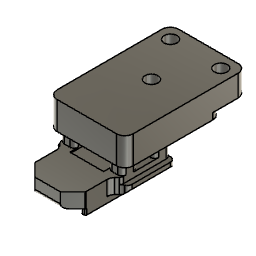
Hybrid_Changer (Autodesk Fusion 360 archive; units mm, degrees)
design "Heating assembly"
Autodesk Fusion 360 part; units mm, degrees
sketch "Sketch1" plane through (0, 0, 0) normal (0, 0, 1) x (1, 0, 0)
  line L0 (9.04, -14.44) -> (-9.04, -14.44)
  line L1 (-9.04, -14.44) -> (-9.04, 14.44)
  line L2 (-9.04, 14.44) -> (9.04, 14.44)
  line L3 (9.04, 14.44) -> (9.04, -14.44)
  line L4 (9.04, -14.44) -> (-9.04, 14.44) construction
  line L5 (-9.04, -14.44) -> (9.04, 14.44) construction
  dimension "d1" = 18.08
  dimension "d2" = 28.88
  constraint horizontal L0
  constraint perpendicular L0 L1
  constraint parallel L0 L2
  constraint parallel L1 L3
  constraint coincident L4 origin
  constraint coincident L5 origin
  measures "d1" distance of L1.end L2.end
  measures "d2" distance of L0.end L1.end
extrude "Extrude1" add sketch "Sketch1" against normal blind 5.6 makes body 1
sketch "Sketch2" plane through (0, 0, 0) normal (0, 0, 1) x (-1, 0, 0)
  line L0 (-9.04, -14.44) -> (9.04, -14.44)
  line L1 (9.04, -14.44) -> (9.04, 14.44)
  line L2 (9.04, 14.44) -> (-9.04, 14.44)
  line L3 (-9.04, 14.44) -> (-9.04, -14.44)
  circle A0 centre (-5.965, -11.415) radius 1.525
  circle A1 centre (5.965, -11.415) radius 1.525
  line L4 (-7.49, -11.415) -> (-9.04, -11.415) construction
  line L5 (-5.965, -12.94) -> (-5.965, -14.44) construction
  line L6 (7.49, -11.415) -> (9.04, -11.415) construction
  line L7 (5.965, -12.94) -> (5.965, -14.44) construction
  circle A2 centre (0, -7.89) radius 1.75
  line L8 (0, -9.64) -> (0, -14.44) construction
  circle A3 centre (0, -0.915) radius 1.525
  line L9 (0, -2.44) -> (0, -0.915) construction
  circle A4 centre (5.89, 11.44) radius 1.85
  circle A5 centre (5.89, 3.44) radius 1.85
  circle A6 centre (-5.89, 11.44) radius 1.85
  circle A7 centre (-5.89, 3.44) radius 1.85
  line L10 (5.89, 13.29) -> (5.89, 11.44) construction
  line L11 (5.89, 11.44) -> (7.74, 11.44) construction
  line L12 (-5.89, 11.44) -> (-7.74, 11.44) construction
  line L13 (5.89, 3.44) -> (5.89, 5.29) construction
  circle A8 centre (5.89, 11.44) radius 1.25
  circle A9 centre (5.89, 3.44) radius 1.25
  circle A10 centre (-5.89, 3.44) radius 1.25
  circle A11 centre (-5.89, 11.44) radius 1.25
  dimension "d5" = 3.05
  dimension "d6" = 1.55
  dimension "d7" = 1.5
  dimension "d8" = 3.5
  dimension "d9" = 4.8
  dimension "d10" = 12
  dimension "d11" = 3.7
  dimension "d12" = 3.7
  dimension "d13" = 3.7
  dimension "d14" = 3.7
  dimension "d15" = 1.15
  dimension "d16" = 1.3
  dimension "d17" = 1.3
  dimension "d18" = 9.15
  dimension "d22" = 2.5
  constraint equal A0 A1
  constraint horizontal A0.centre A1.centre
  constraint coincident A0 L4.start
  constraint coincident L3 L4.end
  constraint perpendicular L3 L4
  constraint coincident A0 L5.start
  constraint coincident L0 L5.end
  constraint perpendicular L0 L5
  constraint coincident A1 L6.start
  constraint coincident L1 L6.end
  constraint perpendicular L1 L6
  constraint coincident A1 L7.start
  constraint coincident L0 L7.end
  constraint perpendicular L0 L7
  constraint horizontal A1.centre L6.start
  constraint vertical A1.centre L7.start
  constraint vertical A0.centre L5.start
  constraint horizontal A0.centre L4.start
  constraint equal L4 L6
  constraint vertical origin A2.centre
  constraint coincident A2 L8.start
  constraint midpoint L0 L8.end
  constraint vertical A2.centre L8.start
  constraint vertical origin A3.centre
  constraint equal A0 A3
  constraint coincident A3 L9.start
  constraint coincident A3.centre L9.end
  constraint vertical L9
  constraint horizontal A4.centre A6.centre
  constraint vertical A4.centre A5.centre
  constraint vertical A6.centre A7.centre
  constraint horizontal A5.centre A7.centre
  constraint coincident A4 L10.start
  constraint coincident A4.centre L10.end
  constraint coincident A4 L11.end
  constraint perpendicular L10 L11
  constraint coincident A6.centre L12.start
  constraint coincident A6 L12.end
  constraint parallel L11 L12
  constraint vertical L10
  constraint coincident A5.centre L13.start
  constraint coincident A5 L13.end
  constraint vertical L13
  constraint concentric A4 A8
  constraint concentric A5 A9
  constraint concentric A7 A10
  constraint concentric A6 A11
  constraint equal A8 A9
  constraint equal A8 A10
  constraint equal A8 A11
  measures "d5" diameter of A0
  measures "d6" distance of L4.start L4.end
  measures "d7" distance of L5.start L5.end
  measures "d8" diameter of A2
  measures "d9" distance of L8.start L8.end
  measures "d10" distance of L8.end L9.start
  measures "d11" diameter of A4
  measures "d12" diameter of A5
  measures "d13" diameter of A6
  measures "d14" diameter of A7
  measures "d15" distance of L2 L10.start
  measures "d16" distance of L1 L11.end
  measures "d17" distance of L3 L12.end
  measures "d18" distance of L2 L13.end
  measures "d22" diameter of A8
extrude "Extrude2" cut sketch "Sketch2" against normal through all contours A0 | A1 | A2 | A3 | A8 | A9 | A10 | A11 bodies 1
extrude "Extrude3" cut sketch "Sketch2" against normal blind 2.35 contours A4 | A5 | A6 | A7 | A8 | A9 | A10 | A11 bodies 1
sketch "Sketch3" plane through (0, 0, -5.6) normal (0, 0, -1) x (1, 0, 0)
  circle A0 centre (-5.89, 11.44) radius 1.25
  circle A1 centre (0, -7.89) radius 1.75
  circle A2 centre (-5.965, -11.415) radius 1.525
  circle A3 centre (5.89, 11.44) radius 1.25
  circle A4 centre (-5.89, 3.44) radius 1.25
  circle A5 centre (0, -0.915) radius 1.525
  circle A6 centre (5.965, -11.415) radius 1.525
  circle A7 centre (5.89, 3.44) radius 1.25
  line L0 (-9.04, -14.44) -> (9.04, -14.44)
  line L1 (9.04, -14.44) -> (9.04, 14.44)
  line L2 (9.04, 14.44) -> (-9.04, 14.44)
  line L3 (-9.04, 14.44) -> (-9.04, -14.44)
  circle A8 centre (0, -0.915) radius 3
  circle A9 centre (5.965, -11.415) radius 3
  circle A10 centre (-5.965, -11.415) radius 3
  line L4 (5.965, -8.415) -> (9.04, -8.415)
  line L5 (2.965, -11.415) -> (2.965, -14.44)
  line L6 (-2.965, -11.415) -> (-2.965, -14.44)
  line L7 (-5.965, -8.415) -> (-9.04, -8.415)
  dimension "d23" = 6
  dimension "d24" = 6
  dimension "d25" = 6
  constraint concentric A5 A8
  constraint concentric A6 A9
  constraint concentric A2 A10
  constraint coincident A9 L4.start
  constraint coincident L1 L4.end
  constraint perpendicular L1 L4
  constraint coincident A9 L5.start
  constraint coincident L0 L5.end
  constraint perpendicular L0 L5
  constraint coincident A10 L6.start
  constraint coincident L0 L6.end
  constraint perpendicular L0 L6
  constraint coincident L3 L7.end
  constraint perpendicular L3 L7
  constraint vertical A6.centre L4.start
  constraint horizontal A6.centre L5.start
  constraint horizontal A2.centre L6.start
  constraint vertical A2.centre L7.start
  constraint coincident A10 L7.start
  measures "d23" diameter of A8
  measures "d24" diameter of A9
  measures "d25" diameter of A10
extrude "Extrude4" cut sketch "Sketch3" against normal blind 1.5 contours A0 | A1 | A2 | A3 | A4 | A5 | A7 | L0 L3 A10 L6 L7 | L0 L1 A9 L4 L5 | A10 | A9 | A8 bodies 1
fillet "Fillet1" radius 2 6 edges at (-9.04, 14.44, -2.05) (9.04, 14.44, -2.05) (-9.04, -14.44, -2.8) (9.04, -14.44, -2.8) (9.04, 8.415, -4.85) (-9.04, 8.415, -4.85) on bodies 1
sketch "Sketch5" plane through (0, 0, -5.6) normal (0, 0, -1) x (1, 0, 0)
  arc A0 (9.04, 12.44) -> (7.04, 14.44) centre (7.04, 12.44) ccw
  line L0 (7.04, 14.44) -> (-7.04, 14.44)
  arc A1 (-7.04, 14.44) -> (-9.04, 12.44) centre (-7.04, 12.44) ccw
  line L1 (-9.04, 12.44) -> (-9.04, -6.415)
  arc A2 (-2.965, -11.415) -> (-5.965, -8.415) centre (-5.965, -11.415) ccw
  line L2 (-2.965, -11.415) -> (-2.965, -14.44)
  line L3 (-2.965, -14.44) -> (2.965, -14.44)
  line L4 (2.965, -14.44) -> (2.965, -11.415)
  arc A3 (5.965, -8.415) -> (2.965, -11.415) centre (5.965, -11.415) ccw
  line L5 (9.04, -6.415) -> (9.04, 12.44)
  circle A4 centre (0, -0.915) radius 3
  circle A5 centre (-5.89, 11.44) radius 1.25
  circle A6 centre (0, -7.89) radius 1.75
  circle A7 centre (5.89, 11.44) radius 1.25
  circle A8 centre (-5.89, 3.44) radius 1.25
  circle A9 centre (5.89, 3.44) radius 1.25
  line L6 (7.34, 1.94) -> (-7.34, 1.94)
  line L7 (-7.34, 1.94) -> (-7.34, 13.44)
  line L8 (-7.34, 13.44) -> (7.34, 13.44)
  line L9 (7.34, 13.44) -> (7.34, 1.94)
  line L10 (7.34, 1.94) -> (-7.34, 13.44) construction
  line L11 (-7.34, 1.94) -> (7.34, 13.44) construction
  line L12 (5.965, -8.415) -> (7.04, -8.415)
  line L13 (-7.04, -8.415) -> (-5.965, -8.415)
  arc A10 (-9.04, -6.415) -> (-7.04, -8.415) centre (-7.04, -6.415) ccw
  arc A11 (7.04, -8.415) -> (9.04, -6.415) centre (7.04, -6.415) ccw
  point P0 (0, 7.69)
  dimension "d33" = 1.7
  dimension "d34" = 1
  dimension "d35" = 12.5
  constraint horizontal L6
  constraint perpendicular L6 L7
  constraint parallel L6 L8
  constraint parallel L7 L9
  constraint coincident L10 P0
  constraint coincident L11 P0
  constraint vertical origin P0
  measures "d33" distance of L5 L9
  measures "d34" distance of L0 L8
  measures "d35" distance of L0 L6
extrude "Extrude5" add sketch "Sketch5" along normal blind 6.2 separate body contours A4 L6 | A4 L6 L7 L8 L9 picked at (0.1862, 1.9708) makes body 2
sketch "Sketch6" plane through (0, 0, -11.8) normal (0, 0, -1) x (1, 0, 0)
  circle A0 centre (5.89, 11.44) radius 1.25
  circle A1 centre (-5.89, 3.44) radius 1.25
  circle A2 centre (5.89, 3.44) radius 1.25
  circle A3 centre (-5.89, 11.44) radius 1.25
  line L0 (7.34, 13.44) -> (-7.34, 13.44)
  line L1 (-7.34, 13.44) -> (-7.34, 1.94)
  line L2 (-7.34, 1.94) -> (7.34, 1.94)
  line L3 (7.34, 1.94) -> (7.34, 13.44)
  line L4 (8.5, 1.94) -> (-8.5, 1.94)
  line L5 (-8.5, 1.94) -> (-8.5, 12.94)
  line L6 (-8.5, 12.94) -> (8.5, 12.94)
  line L7 (8.5, 12.94) -> (8.5, 1.94)
  line L8 (8.5, 1.94) -> (-8.5, 12.94) construction
  line L9 (-8.5, 1.94) -> (8.5, 12.94) construction
  line L10 (8.5, 12.94) -> (7.34, 13.44)
  line L11 (-7.34, 13.44) -> (-8.5, 12.94)
  point P0 (0, 7.44)
  dimension "d38" = 17
  dimension "d39" = 11
  constraint horizontal L4
  constraint perpendicular L4 L5
  constraint parallel L4 L6
  constraint parallel L5 L7
  constraint coincident L8 P0
  constraint coincident L9 P0
  constraint vertical origin P0
  constraint coincident L2.end L4
  constraint coincident L0.start L3.end
  constraint coincident L0.end L1.start
  measures "d38" distance of L5.end L6.end
  measures "d39" distance of L4.end L5.end
extrude "Extrude6" add sketch "Sketch6" against normal blind 2 contours A0 | A1 | A2 | A3 | L3 L6 L10 | L1 L6 L11 | L3 L4 L6 L7 | L1 L2 L3 L4 L6 | L1 L4 L5 L6 bodies 2
sketch "Sketch7" plane through (0, 0, -11.8) normal (0, 0, -1) x (1, 0, 0)
  line L0 (7.34, 13.44) -> (-7.34, 13.44)
  line L1 (-8.5, 12.94) -> (-8.5, 1.94)
  line L2 (-8.5, 1.94) -> (8.5, 1.94)
  line L3 (8.5, 1.94) -> (8.5, 12.94)
  line L4 (6.025, 13.44) -> (-6.025, 13.44)
  line L5 (-6.025, 13.44) -> (-6.025, 23.74)
  line L6 (-6.025, 23.74) -> (6.025, 23.74)
  line L7 (6.025, 23.74) -> (6.025, 13.44)
  line L8 (0, 23.74) -> (0, 0) construction
  line L9 (8.5, 12.94) -> (7.34, 13.44)
  line L10 (-7.34, 13.44) -> (-8.5, 12.94)
  line L11 (7.34, 13.44) -> (6.025, 14.94)
  line L12 (-6.025, 14.94) -> (-7.34, 13.44)
  dimension "d42" = 12.05
  dimension "d43" = 10.3
  dimension "d70" = 1.5
  constraint horizontal L4
  constraint vertical L5
  constraint horizontal L6
  constraint vertical L7
  constraint coincident L0 L4.start
  constraint midpoint L6 L8.start
  constraint coincident L8.end origin
  constraint vertical L8
  constraint coincident L0.start L9.end
  constraint coincident L7 L11.end
  constraint coincident L5 L12.start
  constraint coincident L0.end L10.start
  constraint horizontal L11.end L12.start
  measures "d42" distance of L4.start L4.end
  measures "d43" distance of L4.start L6.end
  measures "d70" distance of L4.start L11.end
extrude "Extrude7" add sketch "Sketch7" against normal blind 3.5 contours L0 L7 L11 | L0 L4 L5 L6 L7 | L0 L5 L12 bodies 2
chamfer "Chamfer3" distance 3 angle 45 2 edges at (6.025, -23.74, -10.05) (-6.025, -23.74, -10.05) on bodies 2
sketch "Sketch10" plane through (0, 0, -11.8) normal (0, 0, -1) x (1, 0, 0)
  line L0 (-6.025, 20.74) -> (-6.025, 14.94)
  line L1 (-8.5, 12.94) -> (-8.5, 1.94)
  line L2 (-8.5, 1.94) -> (8.5, 1.94)
  line L3 (8.5, 1.94) -> (8.5, 12.94)
  line L4 (6.025, 14.94) -> (6.025, 20.74)
  line L5 (3.025, 23.74) -> (-3.025, 23.74)
  line L6 (6.025, 20.74) -> (5.025, 20.74)
  line L7 (5.025, 20.74) -> (5.025, 1.94)
  line L8 (5.025, 1.94) -> (6.025, 1.94)
  line L9 (6.025, 1.94) -> (6.025, 20.74)
  line L10 (-6.025, 20.74) -> (-5.025, 20.74)
  line L11 (-5.025, 20.74) -> (-5.025, 1.94)
  line L12 (-5.025, 1.94) -> (-6.025, 1.94)
  line L13 (-6.025, 1.94) -> (-6.025, 3.24)
  line L14 (-6.525, 3.74) -> (-7.025, 3.74)
  line L15 (-7.025, 3.74) -> (-7.025, 11.64)
  line L16 (-7.025, 11.64) -> (-6.525, 11.64)
  line L17 (-6.025, 11.64) -> (-6.025, 3.74)
  arc A0 (-6.025, 3.24) -> (-6.525, 3.74) centre (-6.525, 3.24) ccw
  line L18 (-6.025, 14.94) -> (-6.025, 12.14)
  arc A1 (-6.525, 11.64) -> (-6.025, 12.14) centre (-6.525, 12.14) ccw
  line L19 (-3.025, 23.74) -> (-6.025, 20.74)
  line L20 (6.025, 20.74) -> (3.025, 23.74)
  line L21 (7.34, 13.44) -> (8.5, 12.94)
  line L22 (8.5, 12.94) -> (7.34, 13.44)
  line L23 (-7.34, 13.44) -> (-8.5, 12.94)
  line L24 (-6.025, 14.94) -> (-7.34, 13.44)
  line L25 (7.34, 13.44) -> (6.025, 14.94)
  dimension "d55" = 1
  dimension "d56" = 1
  dimension "d60" = 1
  dimension "d61" = 1.8
  dimension "d63" = 0.5
  dimension "d64" = 0.5
  constraint horizontal L6
  constraint vertical L7
  constraint horizontal L8
  constraint vertical L9
  constraint coincident L4.end L6.start
  constraint horizontal L10
  constraint vertical L11
  constraint horizontal L12
  constraint vertical L13
  constraint coincident L2 L11.end
  constraint coincident L0.start L10.start
  constraint coincident L2 L7.end
  constraint horizontal L14
  constraint vertical L15
  constraint horizontal L16
  constraint vertical L17
  constraint coincident L13 L17.end
  constraint coincident L17.end L14
  constraint coincident L0.start L13
  constraint tangent L14 A0
  constraint tangent L13 A0
  constraint coincident L0.end L18.start
  constraint coincident L17.start L16
  constraint coincident L17.start L18
  constraint tangent L16 A1
  constraint tangent L18 A1
  constraint coincident L21.start L22.end
  constraint coincident L3.end L21.end
  measures "d55" distance of L4.end L6.end
  measures "d56" distance of L0.start L10.end
  measures "d60" distance of L17.end L14.end
  measures "d61" distance of L2 L14
  measures "d63" radius of A0
  measures "d64" radius of A1
extrude "Extrude10" add sketch "Sketch10" along normal blind 1.65 contours L0 L2 L10 L11 L12 L13 L14 L15 L16 A0 L18 A1 | L2 L4 L6 L7 L8 L9 bodies 2
chamfer "Chamfer2" distance 1 angle 45 2 edges at (8.5, -7.44, -11.8) (-8.5, -7.44, -11.8) on bodies 2
sketch "Sketch11" plane through (0, 0, -11.8) normal (0, 0, -1) x (1, 0, 0)
  line L0 (7.5, 1.94) -> (7.5, 13.371)
  line L1 (6.025, 14.94) -> (6.025, 1.94)
  line L2 (6.025, 1.94) -> (7.5, 1.94)
  line L3 (6.025, 1.94) -> (6.025, 20.74)
  line L4 (7.5, 13.371) -> (7.34, 13.44)
  line L5 (7.34, 13.44) -> (6.025, 14.94)
  point P0 (8.5, 12.94)
  point P1 (8.5, 1.94)
fillet "Fillet3" radius 1.15 4 edges at (-8.5, -12.94, -10.3) (8.5, -12.94, -10.3) (8.5, -1.94, -10.3) (-8.5, -1.94, -10.3) on bodies 2
fillet "Fillet4" radius 2 4 edges at (6.025, -14.94, -10.05) (7.34, -13.44, -10.8) (-6.025, -14.94, -10.05) (-7.34, -13.44, -10.8) on bodies 2
sketch "Sketch12" plane through (7.34, 0, 0) normal (1, 0, 0) x (0, 1, 0)
  line L0 (-13.5027, -9.8) -> (-1.94, -9.8)
  line L1 (-1.94, -9.8) -> (-1.94, -5.6)
  line L2 (-1.94, -5.6) -> (-13.44, -5.6)
  line L3 (-13.44, -5.6) -> (-13.44, -8.3)
  line L4 (-13.44, -8.3) -> (-13.5027, -8.3)
  line L5 (-13.5027, -8.3) -> (-13.5027, -9.8)
  line L6 (-5.69, -5.6) -> (-9.69, -5.6)
  line L7 (-9.69, -5.6) -> (-9.69, -8.6)
  line L8 (-9.69, -8.6) -> (-5.69, -8.6)
  line L9 (-5.69, -8.6) -> (-5.69, -5.6)
  point P0 (-7.69, -5.6)
  point P1 (-7.69, -8.6)
  dimension "d73" = 4
  dimension "d74" = 3
  constraint horizontal L6
  constraint vertical L7
  constraint horizontal L8
  constraint vertical L9
  constraint coincident L2 L6.start
  constraint midpoint L2 P0
  constraint midpoint L8 P1
  constraint vertical P0 P1
  measures "d73" distance of L6.start L6.end
  measures "d74" distance of L6.start L8.end
extrude "Extrude11" cut sketch "Sketch12" against normal through all contours L2 L6 L7 L8 L9 bodies 2
sketch "Sketch13" plane through (0, -1.94, 0) normal (0, 1, 0) x (-1, 0, 0)
  line L0 (7.35, -11.8) -> (7.35, -9.8)
  line L1 (7.35, -9.8) -> (7.34, -9.8)
  line L2 (7.34, -9.8) -> (7.34, -5.6)
  line L3 (7.34, -5.6) -> (-7.34, -5.6)
  line L4 (-7.34, -5.6) -> (-7.34, -9.8)
  line L5 (-7.34, -9.8) -> (-7.35, -9.8)
  line L6 (-7.35, -9.8) -> (-7.35, -11.8)
  line L7 (-7.35, -11.8) -> (-6.025, -11.8)
  line L8 (-6.025, -11.8) -> (-6.025, -13.45)
  line L9 (-6.025, -13.45) -> (-5.025, -13.45)
  line L10 (-5.025, -13.45) -> (-5.025, -11.8)
  line L11 (-5.025, -11.8) -> (5.025, -11.8)
  line L12 (5.025, -11.8) -> (5.025, -13.45)
  line L13 (5.025, -13.45) -> (6.025, -13.45)
  line L14 (6.025, -13.45) -> (6.025, -11.8)
  line L15 (6.025, -11.8) -> (7.35, -11.8)
  line L16 (4, -5.6) -> (-4, -5.6)
  line L17 (-4, -5.6) -> (-4, -8.6)
  line L18 (-4, -8.6) -> (4, -8.6)
  line L19 (4, -8.6) -> (4, -5.6)
  point P0 (0, -5.6)
  point P1 (0, -8.6)
  dimension "d76" = 8
  dimension "d77" = 3
  constraint horizontal L16
  constraint vertical L17
  constraint horizontal L18
  constraint vertical L19
  constraint coincident L3 L16.start
  constraint midpoint L3 P0
  constraint midpoint L18 P1
  constraint vertical P0 P1
  measures "d76" distance of L16.start L16.end
  measures "d77" distance of L16.start L18.end
extrude "Extrude12" cut sketch "Sketch13" against normal blind 12.5 contours L3 L16 L17 L18 L19 bodies 2
fillet "Fillet5" radius 1 19 edges at (-7.34, -1.94, -7.7) (-7.34, -5.69, -7.1) (-4, -1.94, -7.1) (-4, -5.69, -7.1) (-7.34, -9.69, -7.1) (-4, -9.69, -7.1) (-7.34, -13.44, -6.95) (-4, -13.44, -6.95) (4, -1.94, -7.1) (7.34, -1.94, -7.7) (4, -5.69, -7.1) (7.34, -5.69, -7.1) (4, -9.69, -7.1) (7.34, -9.69, -7.1) (7.34, -13.44, -6.95) (4, -13.44, -6.95) (7.34, -13.5027, -9.05) (-7.34, -13.5027, -9.05) (0, -23.74, -11.8) on bodies 2
fillet "Fillet6" radius 0.25 23 edges at (5.025, -20.74, -12.625) (6.025, -11.34, -13.45) (5.525, -20.74, -13.45) (5.025, -11.34, -13.45) (-5.025, -20.74, -12.625) (-6.025, -20.74, -12.625) (-6.025, -20.74, -10.05) (6.025, -20.74, -12.625) (6.025, -20.74, -10.05) (-5.025, -11.34, -13.45) (-5.525, -20.74, -13.45) (-6.025, -16.44, -13.45) (-6.1714, -11.7864, -13.45) (-6.775, -11.64, -13.45) (-6.775, -3.74, -13.45) (-6.1714, -3.5936, -13.45) (-6.025, -2.59, -13.45) (6.025, -1.94, -12.625) (5.025, -1.94, -12.625) (-6.025, -1.94, -12.625) (-5.025, -1.94, -12.625) (-7.025, -11.64, -12.625) (-7.025, -3.74, -12.625) on bodies 2
sketch "Sketch14" plane through (0, 0, 0) normal (0, 0, 1) x (-1, 0, 0)
  circle A0 centre (5.89, 11.44) radius 1.85
  circle A1 centre (-5.89, 11.44) radius 1.85
  circle A2 centre (5.89, 3.44) radius 1.85
  circle A3 centre (-5.89, 3.44) radius 1.85
  circle A4 centre (0, -7.89) radius 1.75
  circle A5 centre (5.965, -11.415) radius 1.525
  circle A6 centre (0, -0.915) radius 1.525
  circle A7 centre (-5.965, -11.415) radius 1.525
  arc A8 (-7.04, 14.44) -> (-9.04, 12.44) centre (-7.04, 12.44) ccw
  line L0 (-9.04, 12.44) -> (-9.04, -12.44)
  arc A9 (-9.04, -12.44) -> (-7.04, -14.44) centre (-7.04, -12.44) ccw
  line L1 (-7.04, -14.44) -> (7.04, -14.44)
  arc A10 (7.04, -14.44) -> (9.04, -12.44) centre (7.04, -12.44) ccw
  line L2 (9.04, -12.44) -> (9.04, 12.44)
  arc A11 (9.04, 12.44) -> (7.04, 14.44) centre (7.04, 12.44) ccw
  line L3 (7.04, 14.44) -> (-7.04, 14.44)
extrude "Extrude13" add sketch "Sketch14" along normal blind 5 separate body makes body 3
sketch "Sketch15" plane through (0, 0, 5) normal (0, 0, 1) x (-1, 0, 0)
  circle A0 centre (5.89, 11.44) radius 1.85
  circle A1 centre (5.89, 3.44) radius 1.85
  circle A2 centre (-5.89, 11.44) radius 1.85
  circle A3 centre (-5.89, 3.44) radius 1.85
  circle A4 centre (0, -0.915) radius 1.525
  circle A5 centre (0, -7.89) radius 1.75
  circle A6 centre (-5.965, -11.415) radius 1.525
  circle A7 centre (5.965, -11.415) radius 1.525
  line L0 (7.04, 14.44) -> (-7.04, 14.44)
  arc A8 (-7.04, 14.44) -> (-9.04, 12.44) centre (-7.04, 12.44) ccw
  line L1 (-9.04, 12.44) -> (-9.04, -12.44)
  arc A9 (-9.04, -12.44) -> (-7.04, -14.44) centre (-7.04, -12.44) ccw
  line L2 (-7.04, -14.44) -> (7.04, -14.44)
  arc A10 (7.04, -14.44) -> (9.04, -12.44) centre (7.04, -12.44) ccw
  line L3 (9.04, -12.44) -> (9.04, 12.44)
  arc A11 (9.04, 12.44) -> (7.04, 14.44) centre (7.04, 12.44) ccw
  circle A12 centre (5.965, -11.415) radius 2.1
  circle A13 centre (0, -0.915) radius 2.1
  circle A14 centre (-5.965, -11.415) radius 2.1
  dimension "d86" = 4.2
  dimension "d87" = 4.2
  dimension "d88" = 4.2
  constraint concentric A7 A12
  constraint concentric A4 A13
  constraint concentric A6 A14
  measures "d86" diameter of A12
  measures "d87" diameter of A13
  measures "d88" diameter of A14
extrude "Extrude14" cut sketch "Sketch15" against normal blind 11 contours A12 | A13 | A14 bodies 3
copy_body "Body->Comp1" bodies 3 removing the originals makes body 4 in component "Component"
sketch "Sketch16" plane through (0, 0, 0) normal (0, 0, 1) x (-1, 0, 0)
  arc A0 (-7.04, 14.44) -> (-9.04, 12.44) centre (-7.04, 12.44) ccw
  line L0 (-9.04, 12.44) -> (-9.04, -12.44)
  arc A1 (-9.04, -12.44) -> (-7.04, -14.44) centre (-7.04, -12.44) ccw
  line L1 (-7.04, -14.44) -> (7.04, -14.44)
  arc A2 (7.04, -14.44) -> (9.04, -12.44) centre (7.04, -12.44) ccw
  line L2 (9.04, -12.44) -> (9.04, 12.44)
  arc A3 (9.04, 12.44) -> (7.04, 14.44) centre (7.04, 12.44) ccw
  line L3 (7.04, 14.44) -> (-7.04, 14.44)
  circle A4 centre (5.89, 11.44) radius 1.85
  circle A5 centre (-5.89, 11.44) radius 1.85
  circle A6 centre (5.89, 3.44) radius 1.85
  circle A7 centre (-5.89, 3.44) radius 1.85
  circle A8 centre (0, -7.89) radius 1.75
  circle A9 centre (5.965, -11.415) radius 1.525
  circle A10 centre (0, -0.915) radius 1.525
  circle A11 centre (-5.965, -11.415) radius 1.525
extrude "Extrude15" add sketch "Sketch16" along normal blind 1 contours A0 L0 A1 L1 A2 L2 A3 L3 | A4 | A5 | A6 | A7 | A8 bodies 1
sketch "Sketch17" plane through (0, 0, 1) normal (0, 0, 1) x (-1, 0, 0)
  circle A0 centre (0, -0.915) radius 1.525
  circle A1 centre (5.965, -11.415) radius 1.525
  circle A2 centre (-5.965, -11.415) radius 1.525
  line L0 (7.04, 14.44) -> (-7.04, 14.44)
  arc A3 (-7.04, 14.44) -> (-9.04, 12.44) centre (-7.04, 12.44) ccw
  line L1 (-9.04, 12.44) -> (-9.04, -12.44)
  arc A4 (-9.04, -12.44) -> (-7.04, -14.44) centre (-7.04, -12.44) ccw
  line L2 (-7.04, -14.44) -> (7.04, -14.44)
  arc A5 (7.04, -14.44) -> (9.04, -12.44) centre (7.04, -12.44) ccw
  line L3 (9.04, -12.44) -> (9.04, 12.44)
  arc A6 (9.04, 12.44) -> (7.04, 14.44) centre (7.04, 12.44) ccw
component "Component" placed x (1, 0, 0) y (0, 1, 0) z (0, 0, 1) at (0, 0, 0)
equation "d17 = d16"

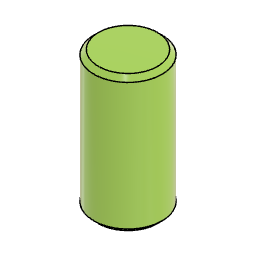
design "Steel_rod_6mm"
Autodesk Fusion 360 part; units mm, degrees
sketch "Sketch1" plane through (0, 0, 0) normal (0, 0, 1) x (1, 0, 0)
  circle A0 centre (0, 0) radius 1.5
  dimension "d1" = 3
  constraint coincident A0.centre origin
  measures "d1" diameter of A0
extrude "Extrude1" add sketch "Sketch1" along normal blind 6 makes body 1
chamfer "Chamfer1" distance 0.2 angle 45 2 edges at (-1.3985, -0.5424, 6) (-1.3985, -0.5424, 0) on bodies 1
copy_body "Body->Comp1" bodies 1 removing the originals makes body 2 in component "Component"
component "Component" placed x (1, 0, 0) y (0, 1, 0) z (0, 0, 1) at (0, 0, 0)
equation "d2 = Length"
equation "Length = 6 mm"

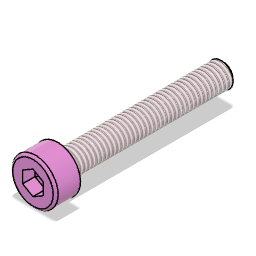
design "Broached Hexagon Socket Head Cap Screw ANSI B18.3.1M - M3x0.5 x 20 Steel Grade 2 Plain"
description: Broached Hexagon Socket Head Cap Screw ANSI B18.3.1M - M3x0.5 x 20
Autodesk Fusion 360 part; units mm, degrees
sketch "Sketch1" plane through (0, 0, 0) normal (0, 1, 0) x (1, 0, 0)
  line L0 (-1.5, 0) -> (-1.5, 20)
  line L1 (-1.5, 20) -> (0, 20)
  line L2 (0, 20) -> (0, -3)
  line L3 (-1.5, 0) -> (-2.75, 0)
  line L4 (-2.75, 0) -> (-2.75, -3)
  line L5 (-2.75, -3) -> (0, -3)
  dimension "d9" = 3
  dimension "d66" = 5.5
  dimension "d68" = 20
  dimension "d79" = 3
  constraint perpendicular L0 L1
  constraint collinear origin L1.end L2.end
  constraint perpendicular L0 L3
  constraint coincident origin L3
  constraint vertical L0
  constraint vertical L2
  constraint parallel L2 L4
  constraint coincident L2 L5.end
  constraint perpendicular L2 L5
  measures "d68" distance of origin L1.end
  measures "d79" distance of L3.end L4.end
revolve "Revolve1" add sketch "Sketch1" angle 360 about axis through (0, 0, -20) along (0, 0, 1)
ref_plane "WorkPlane1" through (0, 0, 3) normal (0, 0, 1) x (1, 0, 0)
sketch "Sketch6" plane through (0, 0, 3) normal (0, 0, 1) x (1, 0, 0)
  line L0 (-1.25, 0) -> (1.25, 0) construction
  line L1 (0, 0) -> (-1.25, 0.7217)
  line L2 (-1.25, -0.7217) -> (-1.25, 0.7217)
  line L3 (-1.25, -0.7217) -> (0, 0)
  dimension "d72" = 2.5
  dimension "d100" = 150
  constraint horizontal L0
  constraint midpoint L1.start L0
  constraint coincident L1.start L3.end
  constraint perpendicular L0 L2
  constraint midpoint L0.start L2
  constraint coincident L1.end L2.end
  measures "d72" distance of L0.start L0.end
  measures "d100" angle of L0 L1
extrude "Extrude1" cut sketch "Sketch6" against normal blind 1.5
pattern_circular "C-Pattern1" count 6 over 360 about axis through (0, 0, 1.75) along (0, 0, 1) of "Extrude1"
extrude "Extrude2" cut 1 faces at (0, -0.4811, 1.5) along direction (0, 0, -1) blind 1.5 draft -85
thread "Thread2" "ANSI Metric M Profile 3.0 M3x0.5 4g6g" major diameter 2.927 minor diameter 2.369 pitch 0.5 angle 60 resizes the face on face at (-1.4981, 0.0748, -6.6667) from (0, 0, -0.9135) to (0, 0, -20)
fillet "Fillet4" radius 0.3 1 edges at (-2.5639, 0.9944, 3)
sketch "Sketch7" plane through (0, 0, 0) normal (0, 1, 0) x (1, 0, 0)
  line L0 (-1.53, 20) -> (-1.53, 19.6933)
  line L1 (-1.53, 19.6933) -> (-1.1933, 20)
  line L2 (0, 20) -> (0, -3)
  line L3 (-1.53, 20) -> (0, 20)
  dimension "d92" = 0.3067
  dimension "d98" = 1.1933
  dimension "d99" = 1.53
  constraint coincident L2.start L3.end
  constraint perpendicular L2 L3
  constraint coincident L1.end L3
  constraint perpendicular L0 L3
  measures "d92" vertical distance of L0.end L1.end
  measures "d98" horizontal distance of origin L1.end
  measures "d99" distance of origin L0
revolve "Revolve3" cut sketch "Sketch7" angle 360 about axis through (0, 0, 1.75) along (0, 0, 1)
equation "d9 = adsk_nomdia"
equation "adsk_nomlen = 20.00 mm"
equation "adsk_headh = 3.00 mm"
equation "adsk_headdia = 5.50 mm"
equation "adsk_nomdia = 3.00 mm"
equation "adsk_waflat = 2.50 mm"
equation "d31 = -adsk_keyend"
equation "adsk_keyend = 1.50 mm"
equation "d66 = adsk_headdia"
equation "d68 = adsk_nomlen"
equation "d71 = adsk_headh"
equation "d72 = adsk_waflat"
equation "d76 = -adsk_keyend"
equation "d79 = adsk_headh"
equation "adsk_thrlen = 19.08655 mm"
equation "d86 = adsk_nomdia * 0.1"
equation "d92 = adsk_startlen"
equation "adsk_startlen = 0.306725 mm"
equation "adsk_endpointdia = 2.38655 mm"
equation "d98 = adsk_endpointdia / 2"
equation "d99 = adsk_nomdia * 0.51"

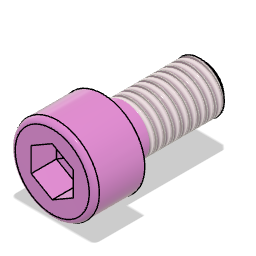
design "Broached Hexagon Socket Head Cap Screw ANSI B18.3.1M - M6x1 x 12 Steel Grade 2 Plain"
description: Broached Hexagon Socket Head Cap Screw ANSI B18.3.1M - M6x1 x 12
Autodesk Fusion 360 part; units mm, degrees
sketch "Sketch1" plane through (0, 0, 0) normal (0, 1, 0) x (1, 0, 0)
  line L0 (-3, 0) -> (-3, 12)
  line L1 (-3, 12) -> (0, 12)
  line L2 (0, 12) -> (0, -6)
  line L3 (-3, 0) -> (-5, 0)
  line L4 (-5, 0) -> (-5, -6)
  line L5 (-5, -6) -> (0, -6)
  dimension "d9" = 6
  dimension "d66" = 10
  dimension "d68" = 12
  dimension "d79" = 6
  constraint perpendicular L0 L1
  constraint collinear origin L1.end L2.end
  constraint perpendicular L0 L3
  constraint coincident origin L3
  constraint vertical L0
  constraint vertical L2
  constraint parallel L2 L4
  constraint coincident L2 L5.end
  constraint perpendicular L2 L5
  measures "d68" distance of origin L1.end
  measures "d79" distance of L3.end L4.end
revolve "Revolve1" add sketch "Sketch1" angle 360 about axis through (0, 0, -12) along (0, 0, 1)
ref_plane "WorkPlane1" through (0, 0, 6) normal (0, 0, 1) x (1, 0, 0)
sketch "Sketch6" plane through (0, 0, 6) normal (0, 0, 1) x (1, 0, 0)
  line L0 (-2.5, 0) -> (2.5, 0) construction
  line L1 (0, 0) -> (-2.5, 1.4434)
  line L2 (-2.5, -1.4434) -> (-2.5, 1.4434)
  line L3 (-2.5, -1.4434) -> (0, 0)
  dimension "d72" = 5
  dimension "d100" = 150
  constraint horizontal L0
  constraint midpoint L1.start L0
  constraint coincident L1.start L3.end
  constraint perpendicular L0 L2
  constraint midpoint L0.start L2
  constraint coincident L1.end L2.end
  measures "d72" distance of L0.start L0.end
  measures "d100" angle of L0 L1
extrude "Extrude1" cut sketch "Sketch6" against normal blind 3
pattern_circular "C-Pattern1" count 6 over 360 about axis through (0, 0, 1.75) along (0, 0, 1) of "Extrude1"
extrude "Extrude2" cut 1 faces at (0.8333, 0.4811, 3) along direction (0, 0, -1) blind 3 draft -85
thread "Thread2" "ANSI Metric M Profile 6.0 M6x1 4g6g" major diameter 5.884 minor diameter 4.764 pitch 1 angle 60 resizes the face on face at (-2.9963, 0.1495, -4) from (0, 0, -2.6135) to (0, 0, -12)
fillet "Fillet4" radius 0.6 1 edges at (-4.6616, 1.8081, 6)
sketch "Sketch7" plane through (0, 0, 0) normal (0, 1, 0) x (1, 0, 0)
  line L0 (-3.06, 12) -> (-3.06, 11.3865)
  line L1 (-3.06, 11.3865) -> (-2.3865, 12)
  line L2 (0, 12) -> (0, -6)
  line L3 (-3.06, 12) -> (0, 12)
  dimension "d92" = 0.6135
  dimension "d98" = 2.3866
  dimension "d99" = 3.06
  constraint coincident L2.start L3.end
  constraint perpendicular L2 L3
  constraint coincident L1.end L3
  constraint perpendicular L0 L3
  measures "d92" vertical distance of L0.end L1.end
  measures "d98" horizontal distance of origin L1.end
  measures "d99" distance of origin L0
revolve "Revolve3" cut sketch "Sketch7" angle 360 about axis through (0, 0, 1.75) along (0, 0, 1)
equation "d9 = adsk_nomdia"
equation "adsk_nomlen = 12.00 mm"
equation "adsk_headh = 6.00 mm"
equation "adsk_headdia = 10.00 mm"
equation "adsk_nomdia = 6.00 mm"
equation "adsk_waflat = 5.00 mm"
equation "d31 = -adsk_keyend"
equation "adsk_keyend = 3.00 mm"
equation "d66 = adsk_headdia"
equation "d68 = adsk_nomlen"
equation "d71 = adsk_headh"
equation "d72 = adsk_waflat"
equation "d76 = -adsk_keyend"
equation "d79 = adsk_headh"
equation "adsk_thrlen = 9.38655 mm"
equation "d86 = adsk_nomdia * 0.1"
equation "d92 = adsk_startlen"
equation "adsk_startlen = 0.61345 mm"
equation "adsk_endpointdia = 4.7731 mm"
equation "d98 = adsk_endpointdia / 2"
equation "d99 = adsk_nomdia * 0.51"

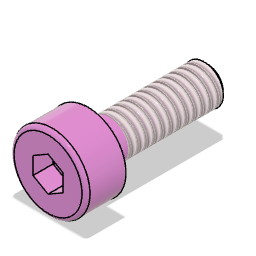
design "Broached Hexagon Socket Head Cap Screw ANSI B18.3.1M - M2x0.4 x 6 Steel Grade 2 Plain"
description: Broached Hexagon Socket Head Cap Screw ANSI B18.3.1M - M2x0.4 x 6
Autodesk Fusion 360 part; units mm, degrees
sketch "Sketch1" plane through (0, 0, 0) normal (0, 1, 0) x (1, 0, 0)
  line L0 (-1, 0) -> (-1, 6)
  line L1 (-1, 6) -> (0, 6)
  line L2 (0, 6) -> (0, -2)
  line L3 (-1, 0) -> (-1.9, 0)
  line L4 (-1.9, 0) -> (-1.9, -2)
  line L5 (-1.9, -2) -> (0, -2)
  dimension "d9" = 2
  dimension "d66" = 3.8
  dimension "d68" = 6
  dimension "d79" = 2
  constraint perpendicular L0 L1
  constraint collinear origin L1.end L2.end
  constraint perpendicular L0 L3
  constraint coincident origin L3
  constraint vertical L0
  constraint vertical L2
  constraint parallel L2 L4
  constraint coincident L2 L5.end
  constraint perpendicular L2 L5
  measures "d68" distance of origin L1.end
  measures "d79" distance of L3.end L4.end
revolve "Revolve1" add sketch "Sketch1" angle 360 about axis through (0, 0, -6) along (0, 0, 1)
ref_plane "WorkPlane1" through (0, 0, 2) normal (0, 0, 1) x (1, 0, 0)
sketch "Sketch6" plane through (0, 0, 2) normal (0, 0, 1) x (1, 0, 0)
  line L0 (-0.75, 0) -> (0.75, 0) construction
  line L1 (0, 0) -> (-0.75, 0.433)
  line L2 (-0.75, -0.433) -> (-0.75, 0.433)
  line L3 (-0.75, -0.433) -> (0, 0)
  dimension "d72" = 1.5
  dimension "d100" = 150
  constraint horizontal L0
  constraint midpoint L1.start L0
  constraint coincident L1.start L3.end
  constraint perpendicular L0 L2
  constraint midpoint L0.start L2
  constraint coincident L1.end L2.end
  measures "d72" distance of L0.start L0.end
  measures "d100" angle of L0 L1
extrude "Extrude1" cut sketch "Sketch6" against normal blind 1
pattern_circular "C-Pattern1" count 6 over 360 about axis through (0, 0, 1.75) along (0, 0, 1) of "Extrude1"
extrude "Extrude2" cut 1 faces at (0, 0.2887, 1) along direction (0, 0, -1) blind 1 draft -85
thread "Thread2" "ANSI Metric M Profile 2.0 M2x0.4 4g6g" major diameter 1.9335 minor diameter 1.4905 pitch 0.4 angle 60 resizes the face on face at (-0.995, 0.0996, -2) from (0, 0, -1.0454) to (0, 0, -6)
fillet "Fillet4" radius 0.2 1 edges at (-1.7714, 0.6871, 2)
sketch "Sketch7" plane through (0, 0, 0) normal (0, 1, 0) x (1, 0, 0)
  line L0 (-1.02, 6) -> (-1.02, 5.7546)
  line L1 (-1.02, 5.7546) -> (-0.7546, 6)
  line L2 (0, 6) -> (0, -2)
  line L3 (-1.02, 6) -> (0, 6)
  dimension "d92" = 0.2454
  dimension "d98" = 0.7546
  dimension "d99" = 1.02
  constraint coincident L2.start L3.end
  constraint perpendicular L2 L3
  constraint coincident L1.end L3
  constraint perpendicular L0 L3
  measures "d92" vertical distance of L0.end L1.end
  measures "d98" horizontal distance of origin L1.end
  measures "d99" distance of origin L0
revolve "Revolve3" cut sketch "Sketch7" angle 360 about axis through (0, 0, 1.75) along (0, 0, 1)
equation "d9 = adsk_nomdia"
equation "adsk_nomlen = 6.00 mm"
equation "adsk_headh = 2.00 mm"
equation "adsk_headdia = 3.80 mm"
equation "adsk_nomdia = 2.00 mm"
equation "adsk_waflat = 1.50 mm"
equation "d31 = -adsk_keyend"
equation "adsk_keyend = 1.00 mm"
equation "d66 = adsk_headdia"
equation "d68 = adsk_nomlen"
equation "d71 = adsk_headh"
equation "d72 = adsk_waflat"
equation "d76 = -adsk_keyend"
equation "d79 = adsk_headh"
equation "adsk_thrlen = 4.95462 mm"
equation "d86 = adsk_nomdia * 0.1"
equation "d92 = adsk_startlen"
equation "adsk_startlen = 0.24538 mm"
equation "adsk_endpointdia = 1.50924 mm"
equation "d98 = adsk_endpointdia / 2"
equation "d99 = adsk_nomdia * 0.51"

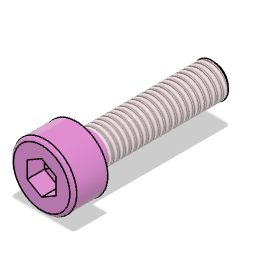
design "Broached Hexagon Socket Head Cap Screw ANSI B18.3.1M - M3x0.5 x 12 Steel Grade 2 Black"
description: Broached Hexagon Socket Head Cap Screw ANSI B18.3.1M - M3x0.5 x 12
Autodesk Fusion 360 part; units mm, degrees
sketch "Sketch1" plane through (0, 0, 0) normal (0, 1, 0) x (1, 0, 0)
  line L0 (-1.5, 0) -> (-1.5, 12)
  line L1 (-1.5, 12) -> (0, 12)
  line L2 (0, 12) -> (0, -3)
  line L3 (-1.5, 0) -> (-2.75, 0)
  line L4 (-2.75, 0) -> (-2.75, -3)
  line L5 (-2.75, -3) -> (0, -3)
  dimension "d9" = 3
  dimension "d66" = 5.5
  dimension "d68" = 12
  dimension "d79" = 3
  constraint perpendicular L0 L1
  constraint collinear origin L1.end L2.end
  constraint perpendicular L0 L3
  constraint coincident origin L3
  constraint vertical L0
  constraint vertical L2
  constraint parallel L2 L4
  constraint coincident L2 L5.end
  constraint perpendicular L2 L5
  measures "d68" distance of origin L1.end
  measures "d79" distance of L3.end L4.end
revolve "Revolve1" add sketch "Sketch1" angle 360 about axis through (0, 0, -12) along (0, 0, 1)
ref_plane "WorkPlane1" through (0, 0, 3) normal (0, 0, 1) x (1, 0, 0)
sketch "Sketch6" plane through (0, 0, 3) normal (0, 0, 1) x (1, 0, 0)
  line L0 (-1.25, 0) -> (1.25, 0) construction
  line L1 (0, 0) -> (-1.25, 0.7217)
  line L2 (-1.25, -0.7217) -> (-1.25, 0.7217)
  line L3 (-1.25, -0.7217) -> (0, 0)
  dimension "d72" = 2.5
  dimension "d100" = 150
  constraint horizontal L0
  constraint midpoint L1.start L0
  constraint coincident L1.start L3.end
  constraint perpendicular L0 L2
  constraint midpoint L0.start L2
  constraint coincident L1.end L2.end
  measures "d72" distance of L0.start L0.end
  measures "d100" angle of L0 L1
extrude "Extrude1" cut sketch "Sketch6" against normal blind 1.5
pattern_circular "C-Pattern1" count 6 over 360 about axis through (0, 0, 1.75) along (0, 0, 1) of "Extrude1"
extrude "Extrude2" cut 1 faces at (0, -0.4811, 1.5) along direction (0, 0, -1) blind 1.5 draft -85
thread "Thread2" "ANSI Metric M Profile 3.0 M3x0.5 4g6g" major diameter 2.927 minor diameter 2.369 pitch 0.5 angle 60 resizes the face on face at (-1.4981, 0.0748, -4) from (0, 0, -1.3067) to (0, 0, -12)
fillet "Fillet4" radius 0.3 1 edges at (-2.5639, 0.9944, 3)
sketch "Sketch7" plane through (0, 0, 0) normal (0, 1, 0) x (1, 0, 0)
  line L0 (-1.53, 12) -> (-1.53, 11.6933)
  line L1 (-1.53, 11.6933) -> (-1.1933, 12)
  line L2 (0, 12) -> (0, -3)
  line L3 (-1.53, 12) -> (0, 12)
  dimension "d92" = 0.3067
  dimension "d98" = 1.1933
  dimension "d99" = 1.53
  constraint coincident L2.start L3.end
  constraint perpendicular L2 L3
  constraint coincident L1.end L3
  constraint perpendicular L0 L3
  measures "d92" vertical distance of L0.end L1.end
  measures "d98" horizontal distance of origin L1.end
  measures "d99" distance of origin L0
revolve "Revolve3" cut sketch "Sketch7" angle 360 about axis through (0, 0, 1.75) along (0, 0, 1)
equation "d9 = adsk_nomdia"
equation "adsk_nomlen = 12.00 mm"
equation "adsk_headh = 3.00 mm"
equation "adsk_headdia = 5.50 mm"
equation "adsk_nomdia = 3.00 mm"
equation "adsk_waflat = 2.50 mm"
equation "d31 = -adsk_keyend"
equation "adsk_keyend = 1.50 mm"
equation "d66 = adsk_headdia"
equation "d68 = adsk_nomlen"
equation "d71 = adsk_headh"
equation "d72 = adsk_waflat"
equation "d76 = -adsk_keyend"
equation "d79 = adsk_headh"
equation "adsk_thrlen = 10.693275 mm"
equation "d86 = adsk_nomdia * 0.1"
equation "d92 = adsk_startlen"
equation "adsk_startlen = 0.306725 mm"
equation "adsk_endpointdia = 2.38655 mm"
equation "d98 = adsk_endpointdia / 2"
equation "d99 = adsk_nomdia * 0.51"

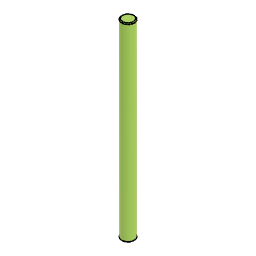
design "Steel_rod_45mm"
Autodesk Fusion 360 part; units mm, degrees
sketch "Sketch1" plane through (0, 0, 0) normal (0, 0, 1) x (1, 0, 0)
  circle A0 centre (0, 0) radius 1.5
  dimension "d1" = 3
  constraint coincident A0.centre origin
  measures "d1" diameter of A0
extrude "Extrude1" add sketch "Sketch1" along normal blind 45 makes body 1
chamfer "Chamfer1" distance 0.2 angle 45 2 edges at (-1.3985, -0.5424, 45) (-1.3985, -0.5424, 0) on bodies 1
copy_body "Body->Comp1" bodies 1 removing the originals makes body 2 in component "Component"
component "Component" placed x (1, 0, 0) y (0, 1, 0) z (0, 0, 1) at (0, 0, 0)
equation "d2 = Length"
equation "Length = 45 mm"

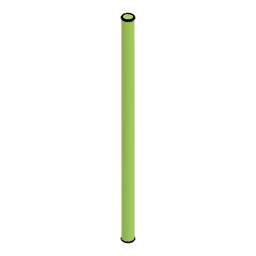
design "Steel_rod_60.5mm"
Autodesk Fusion 360 part; units mm, degrees
sketch "Sketch1" plane through (0, 0, 0) normal (0, 0, 1) x (1, 0, 0)
  circle A0 centre (0, 0) radius 1.5
  dimension "d1" = 3
  constraint coincident A0.centre origin
  measures "d1" diameter of A0
extrude "Extrude1" add sketch "Sketch1" along normal blind 60.5 makes body 1
chamfer "Chamfer1" distance 0.2 angle 45 2 edges at (-1.3985, -0.5424, 60.5) (-1.3985, -0.5424, 0) on bodies 1
copy_body "Body->Comp1" bodies 1 removing the originals makes body 2 in component "Component"
component "Component" placed x (1, 0, 0) y (0, 1, 0) z (0, 0, 1) at (0, 0, 0)
equation "d2 = Length"
equation "Length = 60.5 mm"

design "3030 Extrusion"
Autodesk Fusion 360 part; units mm, degrees
sketch "Sketch1" plane through (0, 0, 0) normal (0, 0, 1) x (1, 0, 0)
  line L0 (270.6, 522.1547) -> (270.6, 519.5346)
  line L1 (259.4, 512.9346) -> (297.4, 512.9346)
  line L2 (263, 528.2346) -> (266, 528.2346)
  line L3 (266, 528.2346) -> (266, 524.1346)
  line L4 (274.1799, 525.7346) -> (270.6, 522.1547)
  line L5 (274.7, 516.5346) -> (273.6, 516.5346)
  line L6 (274.7, 519.5346) -> (274.7, 517.6346)
  line L7 (272.2, 531.8503) -> (272.2843, 531.9346)
  line L8 (265.9, 516.5346) -> (264.4, 516.5346)
  line L9 (272.2, 527.7145) -> (272.2, 531.8503)
  line L10 (263, 535.6346) -> (263, 545.9346)
  arc A0 (263, 517.9346) -> (264.4, 516.5346) centre (264.4, 517.9346) ccw
  line L11 (274.7, 517.6346) -> (274.7, 516.5346)
  line L12 (268.6201, 524.1346) -> (272.2, 527.7145)
  line L13 (273.6, 516.5346) -> (265.9, 516.5346)
  line L14 (266, 535.6346) -> (263, 535.6346)
  line L15 (263, 517.9346) -> (263, 528.2346)
  line L16 (272.2843, 531.9346) -> (272.2, 532.0189)
  line L17 (266, 524.1346) -> (268.6201, 524.1346)
  line L18 (270.6, 519.5346) -> (274.7, 519.5346)
  line L19 (268.6201, 539.7346) -> (266, 539.7346)
  line L20 (266, 539.7346) -> (266, 535.6346)
  line L21 (282.1, 517.6346) -> (282.1, 519.5346)
  line L22 (282.6201, 525.7346) -> (278.4843, 525.7346)
  line L23 (282.1, 516.5346) -> (282.1, 517.6346)
  line L24 (264.4, 547.3346) -> (273.6, 547.3346)
  line L25 (284.5157, 531.9346) -> (284.6, 531.8503)
  line L26 (278.4, 525.8189) -> (278.3157, 525.7346)
  arc A1 (264.4, 547.3346) -> (263, 545.9346) centre (264.4, 545.9346) ccw
  line L27 (274.7, 547.3346) -> (274.7, 546.2346)
  line L28 (274.7, 544.3346) -> (270.6, 544.3346)
  line L29 (278.4843, 525.7346) -> (278.4, 525.8189)
  line L30 (278.3157, 525.7346) -> (274.1799, 525.7346)
  line L31 (274.7, 546.2346) -> (274.7, 544.3346)
  line L32 (273.6, 547.3346) -> (274.7, 547.3346)
  line L33 (272.2, 532.0189) -> (272.2, 536.1547)
  line L34 (270.6, 544.3346) -> (270.6, 541.7145)
  line L35 (270.6, 541.7145) -> (274.1799, 538.1346)
  line L36 (272.2, 536.1547) -> (268.6201, 539.7346)
  line L37 (286.2, 519.5346) -> (286.2, 522.1547)
  line L38 (259.4, 550.9346) -> (259.4, 512.9346)
  line L39 (297.4, 550.9346) -> (259.4, 550.9346)
  line L40 (284.6, 532.0189) -> (284.5157, 531.9346)
  line L41 (282.1, 519.5346) -> (286.2, 519.5346)
  line L42 (274.1799, 538.1346) -> (278.3157, 538.1346)
  line L43 (283.2, 516.5346) -> (282.1, 516.5346)
  line L44 (284.6, 536.1547) -> (284.6, 532.0189)
  line L45 (293.8, 535.6346) -> (290.8, 535.6346)
  line L46 (282.1, 546.2346) -> (282.1, 547.3346)
  line L47 (278.4, 538.0503) -> (278.4843, 538.1346)
  line L48 (282.1, 547.3346) -> (283.2, 547.3346)
  line L49 (288.1799, 524.1346) -> (290.8, 524.1346)
  line L50 (278.4843, 538.1346) -> (282.6201, 538.1346)
  line L51 (290.9, 547.3346) -> (292.4, 547.3346)
  line L52 (292.4, 516.5346) -> (290.9, 516.5346)
  line L53 (282.1, 544.3346) -> (282.1, 546.2346)
  line L54 (293.8, 528.2346) -> (293.8, 517.9346)
  line L55 (290.8, 524.1346) -> (290.8, 528.2346)
  line L56 (286.2, 541.7145) -> (286.2, 544.3346)
  line L57 (284.6, 531.8503) -> (284.6, 527.7145)
  line L58 (290.9, 516.5346) -> (283.2, 516.5346)
  line L59 (290.8, 539.7346) -> (288.1799, 539.7346)
  arc A2 (292.4, 516.5346) -> (293.8, 517.9346) centre (292.4, 517.9346) ccw
  line L60 (282.6201, 538.1346) -> (286.2, 541.7145)
  line L61 (297.4, 512.9346) -> (297.4, 550.9346)
  line L62 (288.1799, 539.7346) -> (284.6, 536.1547)
  line L63 (283.2, 547.3346) -> (290.9, 547.3346)
  line L64 (284.6, 527.7145) -> (288.1799, 524.1346)
  line L65 (286.2, 544.3346) -> (282.1, 544.3346)
  line L66 (290.8, 528.2346) -> (293.8, 528.2346)
  line L67 (278.3157, 538.1346) -> (278.4, 538.0503)
  line L68 (293.8, 545.9346) -> (293.8, 535.6346)
  line L69 (286.2, 522.1547) -> (282.6201, 525.7346)
  line L70 (290.8, 535.6346) -> (290.8, 539.7346)
  arc A3 (293.8, 545.9346) -> (292.4, 547.3346) centre (292.4, 545.9346) ccw
  line L71 (-7.8, 12.4) -> (-7.8, 9.7799)
  line L72 (7.8, -12.4) -> (7.8, -9.7799)
  line L73 (12.4, 7.8) -> (9.7799, 7.8)
  line L74 (-6.2, 0.0843) -> (-6.2, 4.2201)
  line L75 (15.4, -3.7) -> (15.4, -14)
  line L76 (3.7, -15.4) -> (3.7, -14.3)
  line L77 (-4.8, 15.4) -> (-3.7, 15.4)
  line L78 (3.7, 12.4) -> (3.7, 14.3)
  line L79 (15.4, 3.7) -> (12.4, 3.7)
  line L80 (6.2, -0.0843) -> (6.2, -4.2201)
  line L81 (12.5, 15.4) -> (14, 15.4)
  line L82 (14, -15.4) -> (12.5, -15.4)
  line L83 (0.0843, 6.2) -> (4.2201, 6.2)
  line L84 (-3.7, 15.4) -> (-3.7, 14.3)
  line L85 (0, 6.1157) -> (0.0843, 6.2)
  line L86 (4.2201, 6.2) -> (7.8, 9.7799)
  line L87 (-3.7, 14.3) -> (-3.7, 12.4)
  line L88 (12.4, -7.8) -> (12.4, -3.7)
  line L89 (9.7799, -7.8) -> (12.4, -7.8)
  line L90 (7.8, 9.7799) -> (7.8, 12.4)
  line L91 (-3.7, 12.4) -> (-7.8, 12.4)
  arc A4 (15.4, 14) -> (14, 15.4) centre (14, 14) ccw
  line L92 (12.4, 3.7) -> (12.4, 7.8)
  line L93 (3.7, -12.4) -> (7.8, -12.4)
  line L94 (-0.0843, 6.2) -> (0, 6.1157)
  line L95 (6.2, 4.2201) -> (6.2, 0.0843)
  arc A5 (14, -15.4) -> (15.4, -14) centre (14, -14) ccw
  line L96 (12.4, -3.7) -> (15.4, -3.7)
  line L97 (15.4, 14) -> (15.4, 3.7)
  line L98 (3.7, 15.4) -> (4.8, 15.4)
  line L99 (9.7799, 7.8) -> (6.2, 4.2201)
  line L100 (3.7, -14.3) -> (3.7, -12.4)
  line L101 (-7.8, 9.7799) -> (-4.2201, 6.2)
  line L102 (6.2, -4.2201) -> (9.7799, -7.8)
  line L103 (4.8, -15.4) -> (3.7, -15.4)
  line L104 (3.7, 14.3) -> (3.7, 15.4)
  line L105 (7.8, -9.7799) -> (4.2201, -6.2)
  line L106 (7.8, 12.4) -> (3.7, 12.4)
  line L107 (-3.7, -14.3) -> (-3.7, -15.4)
  line L108 (-9.7799, 7.8) -> (-12.4, 7.8)
  line L109 (4.2201, -6.2) -> (0.0843, -6.2)
  line L110 (-4.2201, 6.2) -> (-0.0843, 6.2)
  line L111 (-6.2, -0.0843) -> (-6.1157, 0)
  line L112 (6.2, 0.0843) -> (6.1157, 0)
  line L113 (-3.7, -12.4) -> (-3.7, -14.3)
  line L114 (-15.4, 3.7) -> (-15.4, 14)
  line L115 (-6.1157, 0) -> (-6.2, 0.0843)
  line L116 (-12.4, 3.7) -> (-15.4, 3.7)
  line L117 (4.8, 15.4) -> (12.5, 15.4)
  line L118 (-4.8, -15.4) -> (-12.5, -15.4)
  line L119 (-12.4, 7.8) -> (-12.4, 3.7)
  arc A6 (-14, 15.4) -> (-15.4, 14) centre (-14, 14) ccw
  line L120 (-6.2, 4.2201) -> (-9.7799, 7.8)
  line L121 (6.1157, 0) -> (6.2, -0.0843)
  line L122 (12.5, -15.4) -> (4.8, -15.4)
  line L123 (-14, 15.4) -> (-4.8, 15.4)
  line L124 (-4.2201, -6.2) -> (-7.8, -9.7799)
  line L125 (-3.7, -15.4) -> (-4.8, -15.4)
  line L126 (-9.7799, -7.8) -> (-6.2, -4.2201)
  line L127 (-15.4, -14) -> (-15.4, -3.7)
  line L128 (-7.8, -9.7799) -> (-7.8, -12.4)
  line L129 (0, -6.1157) -> (-0.0843, -6.2)
  line L130 (-12.4, -7.8) -> (-9.7799, -7.8)
  line L131 (-15.4, -3.7) -> (-12.4, -3.7)
  line L132 (0.0843, -6.2) -> (0, -6.1157)
  line L133 (-0.0843, -6.2) -> (-4.2201, -6.2)
  line L134 (-12.5, -15.4) -> (-14, -15.4)
  line L135 (-12.4, -3.7) -> (-12.4, -7.8)
  arc A7 (-15.4, -14) -> (-14, -15.4) centre (-14, -14) ccw
  line L136 (-6.2, -4.2201) -> (-6.2, -0.0843)
  line L137 (-7.8, -12.4) -> (-3.7, -12.4)
  line L138 (-6.1157, 0) -> (6.1157, 0) construction
  line L139 (0, -6.1157) -> (0, 0) construction
  constraint horizontal L138
  constraint vertical L139
  constraint coincident L138 L139.end
extrude "Extrude1" add sketch "Sketch1" along normal blind 527.2 contours L71 L72 L73 L74 L75 L76 L77 L78 L79 L80 L81 L82 L83 L84 L85 L86 L87 L88 L89 L90 L91 A4 L92 L93 L94 L95 A5 L96 L97 L98 L99 L100 L101 L102 L103 L104 L105 L106 L107 L108 L109 L110 L111 L112 L113 L114 L115 L116 L117 L118 L119 A6 L120 L121 L122 L123 L124 L125 L126 L127 L128 L129 L130 L131 L132 L133 L134 L135 A7 L136 L137
